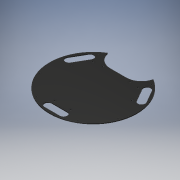
# Autodesk Inventor part: platinetest
Saved by Autodesk Inventor 2018 (Build 220112000, 112)
## iProperties
Created: 2019-03-02
Part Number: platinetest
Material: Kupfer
Document SubType Name: Modeling
Designer: RedBots
Density: 1.88071 g/cm^3
Appearance: Glänzend - schwarz
Mass: 105 g
Surface Area: 582.91 cm^2
Volume: 55.8299 cm^3
Author: RedBots
Autodesk Inventor part; units mm, degrees
ref_plane "YZ Plane" through (0, 0, 0) normal (1, 0, 0) x (0, 1, 0)
ref_plane "XZ Plane" through (0, 0, 0) normal (0, 1, 0) x (-1, 0, 0)
ref_plane "XY Plane" through (0, 0, 0) normal (0, 0, 1) x (1, 0, 0)
sketch "Skizze3" plane through (0, 0, 0) normal (0, 0, 1) x (1, 0, 0)
  arc A0 (-55.0029, 89.4409) -> (55.0029, 89.4409) centre (0, 0) ccw
  line L0 (0, 0) -> (55.0029, 89.4409) construction
  line L1 (0, 0) -> (105, 0) construction
  line L2 (0, 0) -> (-55.0029, 89.4409) construction
  line L3 (-55.0029, 89.4409) -> (-18.8829, 89.4409)
  line L4 (-18.8829, 89.4409) -> (-18.8829, 97.4409)
  arc A1 (-55.0029, 89.4409) -> (-18.8829, 60.4456) centre (-18.8829, 97.4409) ccw
  line L5 (55.0029, 89.4409) -> (18.8829, 89.4409)
  line L6 (18.8829, 89.4409) -> (18.8829, 97.4409)
  arc A2 (18.8839, 60.4456) -> (55.0029, 89.4409) centre (18.8829, 97.4409) ccw
  line L7 (18.8829, 97.4409) -> (18.8839, 60.4456) construction
  line L8 (18.8829, 97.4409) -> (55.0029, 89.4409) construction
  line L9 (-18.8829, 60.4456) -> (18.8839, 60.4456)
  line L10 (0, 0) -> (57.2785, 0) construction
  line L11 (0, 0) -> (57.2785, 0) construction
  line L12 (0, 0) -> (57.279, 0) construction
  line L13 (0, 0) -> (84.4383, 0) construction
  line L14 (0, 0) -> (77.9423, 45)
  line L15 (0, 0) -> (90, 0) construction
  line L16 (0, 0) -> (-77.9423, 45)
  line L17 (0, 0) -> (90, 0) construction
  line L18 (0, 0) -> (0, -90)
  line L19 (0, 0) -> (90, 0) construction
  line L20 (-27.5, -90) -> (27.5, -90) construction
  line L21 (-23, -90) -> (23, -90) construction
  line L22 (-18.5, -90) -> (18.5, -90) construction
  line L23 (-18.5, -99) -> (18.5, -99)
  line L24 (18.5, -81) -> (-18.5, -81)
  arc A3 (-18.5, -81) -> (-18.5, -99) centre (-18.5, -90) ccw
  arc A4 (18.5, -99) -> (18.5, -81) centre (18.5, -90) ccw
  line L25 (87.1923, 28.9785) -> (68.6923, 61.0215) construction
  line L26 (94.9865, 33.4785) -> (76.4865, 65.5215)
  line L27 (60.8981, 56.5215) -> (79.3981, 24.4785)
  arc A5 (79.3981, 24.4785) -> (94.9865, 33.4785) centre (87.1923, 28.9785) ccw
  arc A6 (76.4865, 65.5215) -> (60.8981, 56.5215) centre (68.6923, 61.0215) ccw
  line L28 (-87.1923, 28.9785) -> (-68.6923, 61.0215) construction
  line L29 (-79.3981, 24.4785) -> (-60.8981, 56.5215)
  line L30 (-76.4865, 65.5215) -> (-94.9865, 33.4785)
  arc A7 (-94.9865, 33.4785) -> (-79.3981, 24.4785) centre (-87.1923, 28.9785) ccw
  arc A8 (-60.8981, 56.5215) -> (-76.4865, 65.5215) centre (-68.6923, 61.0215) ccw
  line L31 (-77.9423, 45) -> (-40.9423, 45) construction
  line L32 (-70.1481, 40.5) -> (-15.5885, 9)
  line L33 (-70.1481, 40.5) -> (-60.1481, 40.5) construction
  line L34 (-61.4878, 35.5) -> (-42.4878, 35.5) construction
  line L35 (-61.4878, 35.5) -> (-52.8275, 30.5)
  line L36 (-61.4878, 35.5) -> (-51.4878, 35.5) construction
  line L37 (-52.8275, 30.5) -> (-26.3275, 30.5) construction
  line L38 (-83.3981, 17.5503) -> (-30.3981, 17.5503) construction
  line L39 (70.1481, 40.5) -> (61.4878, 35.5)
  line L40 (70.1481, 40.5) -> (80.1481, 40.5) construction
  line L41 (0, -81) -> (0, -71)
  line L42 (0, -81) -> (10, -81) construction
  line L43 (-70.1481, 40.5) -> (-63.6529, 36.75)
  line L44 (-70.1481, 40.5) -> (-62.6481, 40.5) construction
  line L45 (-70.4077, 10.0503) -> (-83.3981, 17.5503)
  line L46 (-83.3981, 17.5503) -> (-56.8981, 63.4497)
  line L47 (-56.8981, 63.4497) -> (-43.9077, 55.9497)
  line L48 (-43.9077, 55.9497) -> (-70.4077, 10.0503)
  line L49 (-70.4077, 10.0503) -> (-56.8981, 63.4497) construction
  line L50 (-83.3981, 17.5503) -> (-43.9077, 55.9497) construction
  line L51 (70.1481, 40.5) -> (63.6529, 36.75)
  line L52 (70.1481, 40.5) -> (77.6481, 40.5) construction
  line L53 (70.4077, 10.0503) -> (83.3981, 17.5503)
  line L54 (83.3981, 17.5503) -> (56.8981, 63.4497)
  line L55 (56.8981, 63.4497) -> (43.9077, 55.9497)
  line L56 (43.9077, 55.9497) -> (70.4077, 10.0503)
  line L57 (70.4077, 10.0503) -> (56.8981, 63.4497) construction
  line L58 (83.3981, 17.5503) -> (43.9077, 55.9497) construction
  line L59 (0, -81) -> (0, -73.5)
  line L60 (26.5, -66) -> (26.5, -81)
  line L61 (26.5, -81) -> (-26.5, -81)
  line L62 (-26.5, -81) -> (-26.5, -66)
  line L63 (-26.5, -66) -> (26.5, -66)
  line L64 (26.5, -66) -> (-26.5, -81) construction
  line L65 (26.5, -81) -> (-26.5, -66) construction
  line L66 (-63.6529, 36.75) -> (-54.1529, 53.2045)
  line L67 (-63.6529, 36.75) -> (-44.6529, 36.75) construction
  line L68 (-63.6529, 36.75) -> (-73.1529, 20.2955)
  line L69 (-63.6529, 36.75) -> (-44.6529, 36.75) construction
  circle A9 centre (-73.1529, 20.2955) radius 2
  circle A10 centre (-54.1529, 53.2045) radius 2
  line L70 (63.6529, 36.75) -> (54.1529, 53.2045)
  line L71 (63.6529, 36.75) -> (82.6529, 36.75) construction
  circle A11 centre (54.1529, 53.2045) radius 2
  line L72 (63.6529, 36.75) -> (73.1529, 20.2955)
  line L73 (63.6529, 36.75) -> (82.6529, 36.75) construction
  circle A12 centre (73.1529, 20.2955) radius 2
  line L74 (0, -73.5) -> (-19, -73.5)
  line L75 (0, -73.5) -> (19, -73.5) construction
  circle A13 centre (-19, -73.5) radius 2
  line L76 (0, -73.5) -> (19, -73.5)
  line L77 (0, -73.5) -> (19, -73.5) construction
  circle A14 centre (19, -73.5) radius 2
  line L78 (0, 0) -> (97, 0) construction
  line L79 (0, 0) -> (97, 0) construction
  line L80 (0, 0) -> (97, 0) construction
  line L81 (0, 0) -> (97, 0) construction
  line L82 (0, 0) -> (100, 0) construction
  circle A15 centre (-93.9693, -34.202) radius 1.5
  line L83 (0, 0) -> (100, 0) construction
  line L84 (0, 0) -> (100, 0) construction
  line L85 (0, 0) -> (100, 0) construction
  circle A16 centre (-50, -86.6025) radius 1.5
  circle A17 centre (93.9693, -34.202) radius 1.5
  circle A18 centre (50, -86.6025) radius 1.5
  line L86 (0, 0) -> (100, 0) construction
  line L87 (0, 0) -> (100, 0) construction
  circle A19 centre (-64.2788, 76.6044) radius 1.5
  circle A20 centre (64.2788, 76.6044) radius 1.5
  line L88 (-15.5885, 9) -> (-36.3731, 21)
  line L89 (-15.5885, 9) -> (8.4115, 9) construction
  line L90 (-21.0885, -0.5263) -> (-62.6577, 23.4737)
  line L91 (-62.6577, 23.4737) -> (-51.6577, 42.5263)
  line L92 (-51.6577, 42.5263) -> (-10.0885, 18.5263)
  line L93 (-10.0885, 18.5263) -> (-21.0885, -0.5263)
  line L94 (-21.0885, -0.5263) -> (-51.6577, 42.5263) construction
  line L95 (-62.6577, 23.4737) -> (-10.0885, 18.5263) construction
  line L96 (0, 0) -> (36.3731, 21)
  line L97 (0, 0) -> (42, 0) construction
  line L98 (0, 0) -> (0, -42)
  line L99 (0, 0) -> (42, 0) construction
  line L100 (21.0885, -0.5263) -> (62.6577, 23.4737)
  line L101 (62.6577, 23.4737) -> (51.6577, 42.5263)
  line L102 (51.6577, 42.5263) -> (10.0885, 18.5263)
  line L103 (10.0885, 18.5263) -> (21.0885, -0.5263)
  line L104 (21.0885, -0.5263) -> (51.6577, 42.5263) construction
  line L105 (62.6577, 23.4737) -> (10.0885, 18.5263) construction
  line L106 (11, -18) -> (11, -66)
  line L107 (11, -66) -> (-11, -66)
  line L108 (-11, -66) -> (-11, -18)
  line L109 (-11, -18) -> (11, -18)
  line L110 (11, -18) -> (-11, -66) construction
  line L111 (11, -66) -> (-11, -18) construction
  circle A21 centre (-32.5, 56.2917) radius 2
  circle A22 centre (32.5, 56.2917) radius 2
  line L112 (-32.5, 56.2917) -> (32.5, 56.2917) construction
  line L113 (-32.5, 56.2917) -> (0, 0) construction
  line L114 (32.5, 56.2917) -> (0, 0) construction
  line L115 (0, 0) -> (64.2788, 76.6044) construction
  line L116 (0, 0) -> (100, 0) construction
  line L117 (0, 0) -> (-64.2788, 76.6044) construction
  line L118 (0, 0) -> (100, 0) construction
  line L119 (0, 0) -> (-93.9693, -34.202) construction
  line L120 (0, 0) -> (100, 0) construction
  line L121 (0, 0) -> (-50, -86.6025) construction
  line L122 (0, 0) -> (100, 0) construction
  line L123 (0, 0) -> (50, -86.6025) construction
  line L124 (0, 0) -> (100, 0) construction
  line L125 (0, 0) -> (93.9693, -34.202) construction
  line L126 (0, 0) -> (100, 0) construction
  point P0 (57.1729, 88.0696)
  point P1 (69.2286, 39.9691)
  point P2 (73.1257, 42.2191)
  dimension "d22" = 105
  dimension "d23" = 58.41
  dimension "d24" = 63.18
  dimension "d25" = 36.12
  dimension "d26" = 8
  dimension "d27" = 90
  dimension "d28" = 36.12
  dimension "d29" = 8
  dimension "d30" = 90
  dimension "d31" = 77.51
  dimension "d42" = 90
  dimension "d43" = 30
  dimension "d46" = 90
  dimension "d47" = 150
  dimension "d50" = 90
  dimension "d51" = 90
  dimension "d52" = 27.5
  dimension "d54" = 23
  dimension "d56" = 18.5
  dimension "d57" = 18
  dimension "d58" = 18.5
  dimension "d59" = 18
  dimension "d60" = 18.5
  dimension "d61" = 60
  dimension "d62" = 18
  dimension "d63" = 63
  dimension "d82" = 150
  dimension "d85" = 90
  dimension "d87" = 7.5
  dimension "d88" = 30
  dimension "d89" = 53
  dimension "d90" = 7.5
  dimension "d91" = 150
  dimension "d92" = 53
  dimension "d93" = 7.5
  dimension "d94" = 53
  dimension "d95" = 19
  dimension "d96" = 60
  dimension "d97" = 19
  dimension "d98" = 120
  dimension "d99" = 4
  dimension "d100" = 4
  dimension "d101" = 19
  dimension "d102" = 120
  dimension "d103" = 4
  dimension "d104" = 19
  dimension "d105" = 60
  dimension "d106" = 4
  dimension "d107" = 19
  dimension "d108" = 180
  dimension "d109" = 4
  dimension "d110" = 19
  dimension "d111" = 0
  dimension "d112" = 4
  dimension "d127" = 3
  dimension "d134" = 3
  dimension "d135" = 3
  dimension "d136" = 3
  dimension "d140" = 3
  dimension "d141" = 3
  dimension "d142" = 24
  dimension "d143" = 150
  dimension "d144" = 22
  dimension "d145" = 42
  dimension "d146" = 30
  constraints: 222 end point, 75 horizontal, 22 centre point, 20 midpoint, 17 parallel, 16 point on circle, 13 perpendicular, 12 tangent, 10 equal length, 8 coincident, 6 collinear, 5 vertical, 3 point on line, 2 equal radius, 1 horizontal alignment, 31 other
  measures "d23" angle of L1 L0
  measures "d24" angle of L0 L2
  measures "d25" distance of L2.end L3.end
  measures "d26" distance of L3.end L4.end
  measures "d27" angle of L4 L3
  measures "d28" distance of L0.end L5.end
  measures "d29" distance of L5.end L6.end
  measures "d30" angle of L5 L6
  measures "d31" angle of L7 L8
  measures "d43" angle of L15 L14
  measures "d51" angle of L18 L19
  measures "d52" distance of L18.end L20.end
  measures "d54" distance of L18.end L21.end
  measures "d56" distance of L18.end L22.end
  measures "d57" diameter of A4
  measures "d58" distance of L14.end L25.end
  measures "d59" diameter of A6
  measures "d60" distance of L31.start L28.end
  measures "d61" angle of L31 L28
  measures "d62" diameter of A8
  measures "d63" distance of L32.start L32.end
  measures "d82" angle of L39 L40
  measures "d85" angle of L42 L41
  measures "d87" distance of L32.start L43.end
  measures "d88" angle of L43 L44
  measures "d89" distance of L45.end L46.end
  measures "d90" distance of L39.start L51.end
  measures "d91" angle of L51 L52
  measures "d92" distance of L54.end L53.end
  measures "d93" distance of L41.start L59.end
  measures "d94" distance of L60.end L61.end
  measures "d95" distance of L43.end L66.end
  measures "d96" angle of L67 L66
  measures "d97" distance of L43.end L68.end
  measures "d98" angle of L68 L69
  measures "d99" diameter of A9
  measures "d100" diameter of A10
  measures "d101" distance of L51.end L70.end
  measures "d102" angle of L71 L70
  measures "d103" diameter of A11
  measures "d104" distance of L51.end L72.end
  measures "d105" angle of L72 L73
  measures "d106" diameter of A12
  measures "d107" distance of L59.end L74.end
  measures "d108" angle of L74 L75
  measures "d109" diameter of A13
  measures "d110" distance of L59.end L75.end
  measures "d111" distance between parallel lines of L76 L77
  measures "d112" diameter of A14
  measures "d127" diameter of A15
  measures "d134" diameter of A16
  measures "d135" diameter of A17
  measures "d136" diameter of A18
  measures "d140" diameter of A19
  measures "d141" diameter of A20
  measures "d142" distance of L32.end L88.end
  measures "d143" angle of L89 L88
  measures "d144" distance of L90.end L91.end
  measures "d146" angle of L97 L96
extrude "Extrusion3" add sketch "Skizze3" along normal blind 2 contours A1 L9 A2 A0 | L14 L56 L55 L54 L27 | L14 L27 L54 L53 L56 | L56 L100 L103 L14 | L14 L103 L102 L56 | L109 L106 L63 L18 | L18 L63 L108 L109 | L93 L90 L48 L16 | L16 L48 L92 L93 | L48 L16 L29 L46 L47 | L48 L45 L46 L29 L16 | L63 L60 L61 L24 L18 | L18 L24 L61 L62 L63
